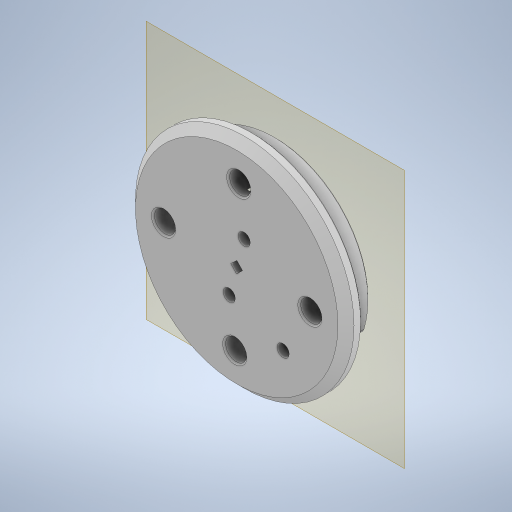
# Autodesk Inventor part: DiffCap
Saved by Autodesk Inventor 2023 (Build 270158000, 158)
## iProperties
Created: 2022-10-30
Part Number: DiffCap
Material: Generic
Document SubType Name: Modeling
Designer: zac-h
Density: 1 g/cm^3
Appearance: Default
Author: zac-h
## iProperties of the stored document DiffCap_3DPrint.ipt
Created: 2022-11-06
Part Number: DiffCap_3DPrint
Material: Generic
Document SubType Name: Modeling
Designer: zac-h
Density: 1 g/cm^3
Appearance: Default
Author: zac-h
Autodesk Inventor part; units mm, degrees
ref_plane "YZ Plane" through (0, 0, 0) normal (1, 0, 0) x (0, 1, 0)
ref_plane "XZ Plane" through (0, 0, 0) normal (0, 1, 0) x (-1, 0, 0)
ref_plane "XY Plane" through (0, 0, 0) normal (0, 0, 1) x (1, 0, 0)
ref_plane "Work Plane1" through (0, 0, 0) normal (0, 0, 1) x (1, 0, 0)
sketch "Sketch1" plane through (0, 0, 0) normal (0, 0, 1) x (1, 0, 0)
  arc A0 (-12.0811, -0.4643) -> (-10.2342, 6.4366) centre (-16.2293, 4.3435) ccw projected
  arc A1 (12.0811, 0.4643) -> (-10.2342, 6.4366) centre (2.9551, 11.0414) ccw projected
  arc A2 (12.0811, 0.4643) -> (10.2342, -6.4366) centre (16.2293, -4.3435) ccw projected
  arc A3 (-12.0811, -0.4643) -> (10.2342, -6.4366) centre (-2.9551, -11.0414) ccw projected
  circle A4 centre (-28.9141, 0.7932) radius 2.413 projected
  circle A5 centre (28.9141, -0.7932) radius 2.413 projected
  circle A6 centre (0.7932, 28.9141) radius 2.413 projected
  circle A7 centre (-0.7932, -28.9141) radius 2.413 projected
  circle A8 centre (0, 0) radius 42.58 projected
  circle A9 centre (0, 0) radius 37.465 construction
  circle A10 centre (0, 0) radius 37.215
  circle A11 centre (18.3343, -19.3686) radius 13.97
  circle A12 centre (-2.9551, -11.0414) radius 13.97
  circle A13 centre (18.3343, -19.3686) radius 2.413 projected
  line L0 (-17.0572, 14.0197) -> (-22.328, 15.5881) projected
  line L1 (-22.328, 15.5881) -> (-23.6052, 20.937) projected
  line L2 (-23.6052, 20.937) -> (-19.6114, 24.7175) projected
  line L3 (-19.6114, 24.7175) -> (-14.3406, 23.1491) projected
  line L4 (-14.3406, 23.1491) -> (-13.0635, 17.8001) projected
  line L5 (-13.0635, 17.8001) -> (-17.0572, 14.0197) projected
  circle A14 centre (-21.1537, -20.0241) radius 2.54 projected
  point P0 (0, 0)
  point P1 (-15.5481, -4.9935)
  point P2 (-12.0811, -0.4643)
  point P3 (10.2342, -6.4366)
  point P4 (10.2342, -6.4366)
  point P5 (-12.0811, -0.4643)
  point P6 (10.6155, -7.7247)
  point P7 (32.2786, -18.5215)
  point P8 (16.7241, -33.2455)
  point P9 (4.7638, -22.6853)
  dimension "d0" = 74.93
  dimension "d1" = 0.25
  dimension "d2" = 27.94
  constraints: 3 centre point, 1 coincident, 3 other
  measures "d0" diameter of A9
  measures "d1" radial gap between concentric circles of A9 A10
  measures "d2" diameter of A11
extrude "Extrusion1" add sketch "Sketch1" along normal blind 11.43 contours A3 A11 A10 A2 A1 A0 | A14
sketch "Sketch2" plane through (0, 0, 11.43) normal (0, 0, 1) x (1, 0, 0)
  arc A0 (10.6155, -7.7247) -> (32.2786, -18.5215) centre (18.3343, -19.3686) ccw projected
  circle A1 centre (0, 0) radius 37.215
  circle A2 centre (0.7932, 28.9141) radius 2.413 projected
  circle A3 centre (0.7932, 28.9141) radius 4.191
  circle A4 centre (-28.9141, 0.7932) radius 4.191
  circle A5 centre (-0.7932, -28.9141) radius 4.191
  circle A6 centre (28.9141, -0.7932) radius 4.191
  arc A7 (4.7638, -22.6853) -> (-12.0811, -0.4643) centre (-2.9551, -11.0414) ccw projected
  circle A8 centre (-2.9551, -11.0414) radius 2.413
  arc A9 (-10.2342, 6.4366) -> (12.0811, 0.4643) centre (2.9551, 11.0414) ccw projected
  circle A10 centre (2.9551, 11.0414) radius 2.413
  circle A11 centre (18.3343, -19.3686) radius 2.413
  dimension "d5" = 8.382
  dimension "d8" = 360
  dimension "d10" = 4.826
  dimension "d11" = 4.826
  dimension "d12" = 4.826
  constraints: 7 centre point, 5 coincident, 12 other
  measures "d5" diameter of A3
  measures "d10" diameter of A8
  measures "d11" diameter of A10
  measures "d12" diameter of A11
extrude "Extrusion2" add sketch "Sketch2" along normal blind 3.81 contours A7 A0 | A1 | A9 A7
sketch "Sketch3" plane through (0, 0, 15.24) normal (0, 0, 1) x (1, 0, 0)
  line L0 (-2.334, 0.064) -> (0.064, 2.334)
  line L1 (0.064, 2.334) -> (2.334, -0.064)
  line L2 (2.334, -0.064) -> (-0.064, -2.334)
  line L3 (-0.064, -2.334) -> (-2.334, 0.064)
  line L4 (-2.334, 0.064) -> (2.334, -0.064) construction
  line L5 (0.064, 2.334) -> (-0.064, -2.334) construction
  circle A0 centre (0, 0) radius 37.215 projected
  circle A1 centre (0.7932, 28.9141) radius 4.191 projected
  circle A2 centre (-0.7932, -28.9141) radius 4.191 projected
  circle A3 centre (18.3343, -19.3686) radius 2.413 projected
  circle A4 centre (2.9551, 11.0414) radius 2.413 projected
  circle A5 centre (-2.9551, -11.0414) radius 2.413 projected
  circle A6 centre (28.9141, -0.7932) radius 4.191 projected
  circle A7 centre (-28.9141, 0.7932) radius 4.191 projected
  circle A8 centre (-0.7932, -28.9141) radius 2.413 projected
  line L6 (28.9141, -0.7932) -> (-0.7932, -28.9141) construction
  line L7 (14.0605, -14.8536) -> (-18.9704, 20.0405) construction
  point P0 (0, 0)
  dimension "d15" = 3.302
  dimension "d16" = 3.302
  constraints: 16 end point, 3 midpoint, 3 perpendicular, 2 parallel
  measures "d15" distance of L1.end L2.end
  measures "d16" distance of L0.end L1.end
extrude "Extrusion3" cut sketch "Sketch3" against normal blind 2.54 contours L0 L1 L2 L3
sketch "Sketch4" plane through (0, 0, 11.43) normal (0, 0, 1) x (1, 0, 0)
  circle A0 centre (-0.7932, -28.9141) radius 2.413 projected
  circle A1 centre (-0.7932, -28.9141) radius 4.191
  circle A2 centre (-28.9141, 0.7932) radius 2.413 projected
  circle A3 centre (-28.9141, 0.7932) radius 4.191
  circle A4 centre (0.7932, 28.9141) radius 2.413 projected
  circle A5 centre (0.7932, 28.9141) radius 4.191
  circle A6 centre (28.9141, -0.7932) radius 2.413 projected
  circle A7 centre (28.9141, -0.7932) radius 4.191
  point P0 (0, 0)
  constraints: 4 centre point, 4 coincident
extrude "Extrusion4" cut sketch "Sketch4" against normal blind 2.54 contours A0 | A1 | A2 | A3 | A4 | A5 | A6 | A7
sketch "Sketch5" plane through (0, 0, 0) normal (0, 0, -1) x (-1, 0, 0)
  circle A0 centre (21.1537, -20.0241) radius 2.54 projected
  point P0 (0, 0)
extrude "Extrusion5" cut sketch "Sketch5" against normal blind 3.81
chamfer "Chamfer1" distance 1.2 angle 45 1 edges at (-18.6137, -20.0241, 0)
fillet "Fillet1" radius 3.175 4 edges at (32.2786, -18.5215, 5.715) (16.7241, -33.2455, 5.715) (4.7638, -22.6853, 5.715) (10.6155, -7.7247, 5.715)
chamfer "Chamfer3" distance 0.6 angle 45 11 edges at (6.5668, 24.5364, 0) (11.195, -0.4733, 0) (10.9575, -5.0176, 0) (7.6262, -28.3406, 0) (23.045, -6.2168, 0) (11.1476, -33.7172, 0) (33.0554, -12.9793, 0) (-25.5835, 27.0267, 0) (4.1911, -24.1493, 0) (-14.9774, -18.1564, 0) (-10.0952, 2.7018, 0)
sketch "Sketch6" plane through (0, 0, 15.24) normal (0, 0, 1) x (1, 0, 0)
  circle A0 centre (0, 0) radius 43.18
  circle A1 centre (0, 0) radius 36.965
  dimension "d33" = 86.36
  constraints: 2 centre point, 2 coincident
  measures "d33" diameter of A0
extrude "Extrusion6" add sketch "Sketch6" against normal blind 6.35
chamfer "Chamfer4" distance 3.175 angle 45 1 edges at (-43.18, 0, 15.24)
chamfer "Chamfer5" distance 0.6 angle 45 1 edges at (-43.18, 0, 8.89)
chamfer "Chamfer6" distance 0.6 angle 45 8 edges at (24.7231, -0.7932, 15.24) (-4.9842, -28.9141, 15.24) (-33.1051, 0.7932, 15.24) (-3.3978, 28.9141, 15.24) (-1.6198, 28.9141, 8.89) (-31.3271, 0.7932, 8.89) (-3.2062, -28.9141, 8.89) (26.5011, -0.7932, 8.89)
body "Solid1"
